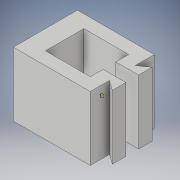
# Autodesk Inventor part: feeding needle holderV2
Saved by Autodesk Inventor 2017 (Build 210142000, 142)
## iProperties
Created: 2017-03-22
Part Number: feeding needle holderV2
Material: Generic
Document SubType Name: Modeling
Designer: Gergely Turi
Density: 1 g/cm^3
Appearance: Default
Author: Gergely Turi
Autodesk Inventor part; units mm, degrees
ref_plane "YZ Plane" through (0, 0, 0) normal (1, 0, 0) x (0, 1, 0)
ref_plane "XZ Plane" through (0, 0, 0) normal (0, 1, 0) x (-1, 0, 0)
ref_plane "XY Plane" through (0, 0, 0) normal (0, 0, 1) x (1, 0, 0)
sketch "Sketch1" plane through (0, 0, 0) normal (0, 1, 0) x (-1, 0, 0)
  line L0 (0, 1) -> (0, 3.1)
  line L1 (0, 3.1) -> (1.55, 2.0147)
  line L2 (0, 3.1) -> (0.6449, 3.1) construction
  line L3 (1.55, 2.0147) -> (1.55, 5)
  line L4 (1.55, 5) -> (1.55, 2.0147)
  line L5 (1.55, 5) -> (13.55, 5)
  line L6 (13.55, 5) -> (13.55, 0.8147)
  line L7 (10.55, 3) -> (10.55, 0.8147)
  line L8 (3.55, 3) -> (3.55, 1)
  line L9 (10.55, 3) -> (3.55, 3)
  line L10 (3.55, 1) -> (0, 1)
  line L11 (0, -1) -> (0, -3.1)
  line L12 (0, -3.1) -> (1.55, -2.0147)
  line L13 (0, -3.1) -> (0.6449, -3.1) construction
  line L14 (1.55, -2.0147) -> (1.55, -5)
  line L15 (1.55, -5) -> (1.55, -2.0147)
  line L16 (1.55, -5) -> (13.55, -5)
  line L17 (13.55, -5) -> (13.55, 0.8147)
  line L18 (10.55, -3) -> (10.55, 0.8147)
  line L19 (3.55, -3) -> (3.55, -1)
  line L20 (10.55, -3) -> (3.55, -3)
  line L21 (3.55, -1) -> (0, -1)
  line L22 (0, 0) -> (8.6928, 0)
  dimension "d3" = 1.55
  dimension "d4" = 12
  dimension "d5" = 3
  dimension "d17" = 6.2
  dimension "d18" = 10
  dimension "d19" = 6
  dimension "d20" = 13.55
  dimension "d21" = 1
  dimension "d22" = 55
  dimension "d26" = 55
  dimension "d27" = 7
  dimension "d28" = 7
  constraints: 46 end point, 5 vertical, 3 horizontal, 3 perpendicular, 1 collinear, 1 parallel, 1 symmetric about line, 3 other
  measures "d3" distance between parallel lines of L0 L3
  measures "d4" distance of L3.end L5.end
  measures "d5" distance between parallel lines of L6 L7
  measures "d17" distance of L0.end L13.start
  measures "d18" distance between parallel lines of L5 L16
  measures "d19" distance between parallel lines of L9 L20
  measures "d20" distance between parallel lines of L11 L17
  measures "d21" distance between parallel lines of L21 L22
  measures "d22" angle of L0 L1
  measures "d26" angle of L11 L12
  measures "d27" distance between parallel lines of L19 L18
  measures "d28" distance between parallel lines of L8 L18
extrude "Extrusion1" add sketch "Sketch1" along normal blind 10
body "Solid1"
